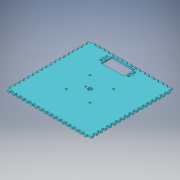
# Autodesk Inventor part: 000.206 - Крышка
Saved by Autodesk Inventor 2019 (Build 230136000, 136)
## iProperties
Created: 2020-02-27
Part Number: 000.206 - Крышка
Material: Типовые
Document SubType Name: Modeling
Designer: Петров Иван
Density: 1 g/cm^3
Appearance: Серо-синий
Author: Петров Иван
Autodesk Inventor part; units mm, degrees
ref_plane "YZ Plane" through (0, 0, 0) normal (1, 0, 0) x (0, 1, 0)
ref_plane "XZ Plane" through (0, 0, 0) normal (0, 1, 0) x (-1, 0, 0)
ref_plane "XY Plane" through (0, 0, 0) normal (0, 0, 1) x (1, 0, 0)
sketch "Эскиз1" plane through (0, 0, 0) normal (0, 1, 0) x (-1, 0, 0)
  line L0 (-72, 72) -> (72, 72)
  line L1 (72, 72) -> (72, -72)
  line L2 (72, -72) -> (-72, -72)
  line L3 (-72, -72) -> (-72, 72)
  line L4 (-72, 72) -> (72, -72) construction
  line L5 (72, 72) -> (-72, -72) construction
  point P0 (0, 0)
  dimension "d0" = 144
  dimension "d1" = 144
  constraints: 12 end point, 2 midpoint, 2 parallel, 1 horizontal, 1 perpendicular
  measures "d0" distance of L1.end L2.end
  measures "d1" distance of L0.end L1.end
extrude "Выдавливание1" add sketch "Эскиз1" along normal blind 3
sketch "Эскиз2" plane through (0, 3, 0) normal (0, 1, 0) x (1, 0, 0)
  line L0 (-72, 72) -> (-72, -72) projected
  line L1 (-72, -72) -> (-68, -72)
  line L2 (-68, -72) -> (-68, -75)
  line L3 (-68, -75) -> (-72, -75)
  line L4 (-72, -75) -> (-72, -72)
  point P0 (0, 0)
  dimension "d5" = 4
  dimension "d6" = 3
  constraints: 8 end point, 2 parallel, 1 horizontal, 1 perpendicular
  measures "d5" distance of L2.end L3.end
  measures "d6" distance of L1.end L2.end
extrude "Выдавливание2" add sketch "Эскиз2" against normal blind 3
pattern_linear "Прямоуг.массив1" count 18 spacing 8 along (1, 0, 0) of "Выдавливание2"
pattern_circular "Круговой массив1" count 4 over 360 about axis through (0, -10, 0) along (0, 1, 0) of "Выдавливание2", "Прямоуг.массив1"
sketch "Эскиз5" plane through (0, 3, 0) normal (0, 1, 0) x (1, 0, 0)
  line L0 (-37.7, 63.75) -> (-37.7, 60.5)
  line L1 (-37.7, 60.5) -> (-30.7, 60.5)
  line L2 (-30.7, 60.5) -> (-30.7, 70)
  line L3 (-30.7, 70) -> (-36.7, 70)
  arc A0 (-36.7, 70) -> (-37.7, 69) centre (-36.7, 69) ccw
  line L4 (-37.7, 69) -> (-37.7, 66.15)
  line L5 (-37.7, 66.15) -> (-36.634, 66.15)
  arc A1 (-36.634, 63.75) -> (-36.634, 66.15) centre (-34.85, 64.95) ccw
  line L6 (-36.634, 63.75) -> (-37.7, 63.75)
  line L7 (-37.7, 59.5) -> (-30.7, 59.5)
  line L8 (-37.7, 59.5) -> (-37.7, 56.25)
  line L9 (-37.7, 56.25) -> (-36.634, 56.25)
  arc A2 (-36.634, 53.85) -> (-36.634, 56.25) centre (-34.85, 55.05) ccw
  line L10 (-36.634, 53.85) -> (-37.7, 53.85)
  line L11 (-37.7, 53.85) -> (-37.7, 51)
  arc A3 (-37.7, 51) -> (-36.7, 50) centre (-36.7, 51) ccw
  line L12 (-36.7, 50) -> (-30.7, 50)
  line L13 (-30.7, 50) -> (-30.7, 59.5)
  line L14 (-37.7, 60.5) -> (-37.7, 59.5)
  line L15 (17, 60.5) -> (17, 59.5)
  line L16 (10, 59.5) -> (17, 59.5)
  line L17 (10, 50) -> (10, 59.5)
  line L18 (16, 50) -> (10, 50)
  arc A4 (16, 50) -> (17, 51) centre (16, 51) ccw
  line L19 (17, 53.85) -> (17, 51)
  line L20 (15.934, 53.85) -> (17, 53.85)
  arc A5 (15.934, 56.25) -> (15.934, 53.85) centre (14.15, 55.05) ccw
  line L21 (17, 56.25) -> (15.934, 56.25)
  line L22 (17, 59.5) -> (17, 56.25)
  line L23 (10, 60.5) -> (10, 70)
  line L24 (10, 60.5) -> (17, 60.5)
  line L25 (17, 63.75) -> (17, 60.5)
  line L26 (15.934, 63.75) -> (17, 63.75)
  arc A6 (15.934, 66.15) -> (15.934, 63.75) centre (14.15, 64.95) ccw
  line L27 (17, 66.15) -> (15.934, 66.15)
  line L28 (17, 69) -> (17, 66.15)
  arc A7 (17, 69) -> (16, 70) centre (16, 69) ccw
  line L29 (10, 70) -> (16, 70)
  line L30 (0, 70) -> (10, 70)
  line L31 (-30.7, 70) -> (0, 70)
  line L32 (-30.7, 50) -> (0, 50)
  line L33 (0, 50) -> (10, 50)
  circle A8 centre (0, 60) radius 5.4
  circle A9 centre (0, 60) radius 6.5
  circle A10 centre (0, 60) radius 1.25
  circle A11 centre (-34.85, 55.05) radius 2.15
  circle A12 centre (-34.85, 64.95) radius 2.15
  circle A13 centre (14.15, 64.95) radius 2.15
  circle A14 centre (14.15, 55.05) radius 2.15
  line L34 (15.934, 53.85) -> (17, 53.85)
  line L35 (17, 56.25) -> (15.934, 56.25)
  line L36 (17, 53.85) -> (17, 56.25)
  line L37 (17, 56.25) -> (17, 66.15)
  line L38 (17, 66.15) -> (15.934, 66.15)
  line L39 (17, 63.75) -> (17, 66.15)
  line L40 (-37.7, 63.75) -> (-37.7, 56.25)
  line L41 (-37.7, 66.15) -> (-37.7, 63.75)
  line L42 (-37.7, 56.25) -> (-36.634, 56.25)
  line L43 (-37.7, 56.25) -> (-37.7, 53.85)
  line L44 (0, 0) -> (0, 70)
  point P0 (-10.35, 50)
  dimension "d29" = 70
  constraints: 90 end point, 16 point on circle, 15 centre point, 4 coincident, 4 vertical, 3 concentric, 1 collinear, 1 perpendicular
  measures "d29" distance of L44.start L44.end
extrude "Выдавливание5" cut sketch "Эскиз5" against normal blind 10 contours L1 L2 L31 L44 A9 L32 L13 L7 L14 | A12 A1 | L30 L23 L24 L15 L16 L17 L33 L44 A9 | A2 A11 | L44 A8 A9 | A9 L44 A8 | L44 A10 A8 | A8 L44 A10 | L44 A10 | A10 L44 | A6 A13 | A14 A5
sketch "Эскиз6" plane through (0, 3, 0) normal (0, 1, 0) x (1, 0, 0)
  arc A0 (-18, 26.5) -> (-26.5, 18) centre (-18, 18) ccw
  line L0 (-26.5, -18) -> (-26.5, 18)
  arc A1 (-26.5, -18) -> (-18, -26.5) centre (-18, -18) ccw
  line L1 (18, -26.5) -> (-18, -26.5)
  arc A2 (18, -26.5) -> (26.5, -18) centre (18, -18) ccw
  line L2 (26.5, 18) -> (26.5, -18)
  arc A3 (26.5, 18) -> (18, 26.5) centre (18, 18) ccw
  line L3 (-18, 26.5) -> (18, 26.5)
  circle A4 centre (-21.2132, 21.2132) radius 1.5
  circle A5 centre (-21.2132, -21.2132) radius 1.5
  circle A6 centre (21.2132, -21.2132) radius 1.5
  circle A7 centre (21.2132, 21.2132) radius 1.5
  circle A8 centre (0, 0) radius 22
  constraints: 9 centre point, 8 end point, 8 point on circle
extrude "Выдавливание6" cut sketch "Эскиз6" against normal blind 10 contours A4 | A5 | A6 | A7
sketch "Эскиз7" plane through (0, 3, 0) normal (0, 1, 0) x (1, 0, 0)
  circle A0 centre (0, 0) radius 5.375
  circle A1 centre (0, 0) radius 3.375
  line L0 (-6.9327, -1) -> (-6.9327, 1)
  line L1 (-6.9327, 1) -> (-6.9327, 1.5)
  line L2 (-8.2327, 1.5) -> (-6.9327, 1.5)
  spline S0 degree 3 poles (-8.308, 1) (-8.3, 1.0653) (-8.2914, 1.1299) (-8.274, 1.2508) (-8.2654, 1.3061) (-8.2506, 1.3973) (-8.2444, 1.4332) (-8.2376, 1.4723) (-8.2358, 1.4829) (-8.2345, 1.49) (-8.2345, 1.4901) (-8.2345, 1.4902) (-8.2339, 1.4935) (-8.2333, 1.4967) (-8.2327, 1.5) knots 0 0 0 0 0.265855 0.265855 0.533308 0.533308 0.789424 0.789424 0.930547 0.930547 0.932946 0.932946 0.932946 1 1 1 1
  ellipse E0 centre (-0.8138, 2.2378) end of major axis (-6.2384, -4.8493) minor radius 6.6293 (-8.308, 1) -> (-8.3138, -1) ccw
  line L3 (-6.9327, -1.5) -> (-8.2327, -1.5)
  line L4 (-6.9327, -1.5) -> (-6.9327, -1)
  spline S1 degree 3 poles (-8.2327, -1.5) (-8.2334, -1.4968) (-8.234, -1.4935) (-8.2347, -1.4903) (-8.2347, -1.4901) (-8.2347, -1.49) (-8.2361, -1.4829) (-8.2382, -1.4724) (-8.2457, -1.4333) (-8.2525, -1.3974) (-8.2687, -1.3062) (-8.278, -1.2509) (-8.2965, -1.1299) (-8.3056, -1.0653) (-8.3138, -1) knots 0 0 0 0 0.066869 0.066869 0.066869 0.069411 0.069411 0.210348 0.210348 0.466356 0.466356 0.734146 0.734146 1 1 1 1
  line L5 (2.8341, 0.75) -> (-2.8341, 0.75)
  line L6 (2.8929, 0.7945) -> (2.8341, 0.75)
  arc A2 (2.8929, 0.7945) -> (2.8468, 0.9465) centre (0, 0) ccw
  line L7 (2.3559, 0.9758) -> (2.8468, 0.9465)
  line L8 (2.6823, 1.3437) -> (2.3559, 0.9758)
  arc A3 (2.6823, 1.3437) -> (2.6074, 1.4837) centre (0, 0) ccw
  line L9 (2.1202, 1.4167) -> (2.6074, 1.4837)
  line L10 (2.3686, 1.8411) -> (2.1202, 1.4167)
  arc A4 (2.3686, 1.8411) -> (2.2678, 1.9639) centre (0, 0) ccw
  line L11 (1.8031, 1.8031) -> (2.2678, 1.9639)
  line L12 (1.9639, 2.2678) -> (1.8031, 1.8031)
  arc A5 (1.9639, 2.2678) -> (1.8411, 2.3686) centre (0, 0) ccw
  line L13 (1.4167, 2.1202) -> (1.8411, 2.3686)
  line L14 (1.4837, 2.6074) -> (1.4167, 2.1202)
  arc A6 (1.4837, 2.6074) -> (1.3437, 2.6823) centre (0, 0) ccw
  line L15 (0.9758, 2.3559) -> (1.3437, 2.6823)
  line L16 (0.9465, 2.8468) -> (0.9758, 2.3559)
  arc A7 (0.9465, 2.8468) -> (0.7945, 2.8929) centre (0, 0) ccw
  line L17 (0.4975, 2.501) -> (0.7945, 2.8929)
  line L18 (0.373, 2.9767) -> (0.4975, 2.501)
  arc A8 (0.373, 2.9767) -> (0.2149, 2.9923) centre (0, 0) ccw
  line L19 (0, 2.55) -> (0.2149, 2.9923)
  line L20 (-0.2149, 2.9923) -> (0, 2.55)
  arc A9 (-0.2149, 2.9923) -> (-0.373, 2.9767) centre (0, 0) ccw
  line L21 (-0.4975, 2.501) -> (-0.373, 2.9767)
  line L22 (-0.7945, 2.8929) -> (-0.4975, 2.501)
  arc A10 (-0.7945, 2.8929) -> (-0.9465, 2.8468) centre (0, 0) ccw
  line L23 (-0.9758, 2.3559) -> (-0.9465, 2.8468)
  line L24 (-1.3437, 2.6823) -> (-0.9758, 2.3559)
  arc A11 (-1.3437, 2.6823) -> (-1.4837, 2.6074) centre (0, 0) ccw
  line L25 (-1.4167, 2.1202) -> (-1.4837, 2.6074)
  line L26 (-1.8411, 2.3686) -> (-1.4167, 2.1202)
  arc A12 (-1.8411, 2.3686) -> (-1.9639, 2.2678) centre (0, 0) ccw
  line L27 (-1.8031, 1.8031) -> (-1.9639, 2.2678)
  line L28 (-2.2678, 1.9639) -> (-1.8031, 1.8031)
  arc A13 (-2.2678, 1.9639) -> (-2.3686, 1.8411) centre (0, 0) ccw
  line L29 (-2.1202, 1.4167) -> (-2.3686, 1.8411)
  line L30 (-2.6074, 1.4837) -> (-2.1202, 1.4167)
  arc A14 (-2.6074, 1.4837) -> (-2.6823, 1.3437) centre (0, 0) ccw
  line L31 (-2.3559, 0.9758) -> (-2.6823, 1.3437)
  line L32 (-2.8468, 0.9465) -> (-2.3559, 0.9758)
  arc A15 (-2.8468, 0.9465) -> (-2.8929, 0.7945) centre (0, 0) ccw
  line L33 (-2.8341, 0.75) -> (-2.8929, 0.7945)
  arc A16 (-2.8929, 0.7945) -> (-2.8929, -0.7945) centre (0, 0) ccw
  line L34 (2.8929, 0.7945) -> (2.8341, 0.75)
  line L35 (2.8341, 0.75) -> (-2.8341, 0.75)
  line L36 (-2.8341, 0.75) -> (-2.8929, 0.7945)
  arc A17 (-2.8929, 0.7945) -> (-2.8929, -0.7945) centre (0, 0) ccw
  line L37 (-2.8929, -0.7945) -> (-2.8341, -0.75)
  line L38 (-2.8341, -0.75) -> (2.8341, -0.75)
  line L39 (2.8341, -0.75) -> (2.8929, -0.7945)
  arc A18 (2.8929, -0.7945) -> (2.8929, 0.7945) centre (0, 0) ccw
  line L40 (-2.8341, -0.75) -> (2.8341, -0.75)
  line L41 (-2.8929, -0.7945) -> (-2.8341, -0.75)
  arc A19 (-2.8929, -0.7945) -> (-2.8468, -0.9465) centre (0, 0) ccw
  line L42 (-2.3559, -0.9758) -> (-2.8468, -0.9465)
  line L43 (-2.6823, -1.3437) -> (-2.3559, -0.9758)
  arc A20 (-2.6823, -1.3437) -> (-2.6074, -1.4837) centre (0, 0) ccw
  line L44 (-2.1202, -1.4167) -> (-2.6074, -1.4837)
  line L45 (-2.3686, -1.8411) -> (-2.1202, -1.4167)
  arc A21 (-2.3686, -1.8411) -> (-2.2678, -1.9639) centre (0, 0) ccw
  line L46 (-1.8031, -1.8031) -> (-2.2678, -1.9639)
  line L47 (-1.9639, -2.2678) -> (-1.8031, -1.8031)
  arc A22 (-1.9639, -2.2678) -> (-1.8411, -2.3686) centre (0, 0) ccw
  line L48 (-1.4167, -2.1202) -> (-1.8411, -2.3686)
  line L49 (-1.4837, -2.6074) -> (-1.4167, -2.1202)
  arc A23 (-1.4837, -2.6074) -> (-1.3437, -2.6823) centre (0, 0) ccw
  line L50 (-0.9758, -2.3559) -> (-1.3437, -2.6823)
  line L51 (-0.9465, -2.8468) -> (-0.9758, -2.3559)
  arc A24 (-0.9465, -2.8468) -> (-0.7945, -2.8929) centre (0, 0) ccw
  line L52 (-0.4975, -2.501) -> (-0.7945, -2.8929)
  line L53 (-0.373, -2.9767) -> (-0.4975, -2.501)
  arc A25 (-0.373, -2.9767) -> (-0.2149, -2.9923) centre (0, 0) ccw
  line L54 (0, -2.55) -> (-0.2149, -2.9923)
  line L55 (0.2149, -2.9923) -> (0, -2.55)
  arc A26 (0.2149, -2.9923) -> (0.373, -2.9767) centre (0, 0) ccw
  line L56 (0.4975, -2.501) -> (0.373, -2.9767)
  line L57 (0.7945, -2.8929) -> (0.4975, -2.501)
  arc A27 (0.7945, -2.8929) -> (0.9465, -2.8468) centre (0, 0) ccw
  line L58 (0.9758, -2.3559) -> (0.9465, -2.8468)
  line L59 (1.3437, -2.6823) -> (0.9758, -2.3559)
  arc A28 (1.3437, -2.6823) -> (1.4837, -2.6074) centre (0, 0) ccw
  line L60 (1.4167, -2.1202) -> (1.4837, -2.6074)
  line L61 (1.8411, -2.3686) -> (1.4167, -2.1202)
  arc A29 (1.8411, -2.3686) -> (1.9639, -2.2678) centre (0, 0) ccw
  line L62 (1.8031, -1.8031) -> (1.9639, -2.2678)
  line L63 (2.2678, -1.9639) -> (1.8031, -1.8031)
  arc A30 (2.2678, -1.9639) -> (2.3686, -1.8411) centre (0, 0) ccw
  line L64 (2.1202, -1.4167) -> (2.3686, -1.8411)
  line L65 (2.6074, -1.4837) -> (2.1202, -1.4167)
  arc A31 (2.6074, -1.4837) -> (2.6823, -1.3437) centre (0, 0) ccw
  line L66 (2.3559, -0.9758) -> (2.6823, -1.3437)
  line L67 (2.8468, -0.9465) -> (2.3559, -0.9758)
  arc A32 (2.8468, -0.9465) -> (2.8929, -0.7945) centre (0, 0) ccw
  line L68 (2.8341, -0.75) -> (2.8929, -0.7945)
  constraints: 138 end point, 62 point on circle, 33 centre point, 8 other
extrude "Выдавливание7" cut sketch "Эскиз7" against normal blind 10 contours A1 | L4 L3 S1 E0 S0 L2 L1 L0 | L6 A18 L39 L38 L37 A16 L33 L5 | L5 L33 A15 L32 L31 A14 L30 L29 A13 L28 L27 A12 L26 L25 A11 L24 L23 A10 L22 L21 A9 L20 L19 A8 L18 L17 A7 L16 L15 A6 L14 L13 A5 L12 L11 A4 L10 L9 A3 L8 L7 A2 L6 | A32 L67 L66 A31 L65 L64 A30 L63 L62 A29 L61 L60 A28 L59 L58 A27 L57 L56 A26 L55 L54 A25 L53 L52 A24 L51 L50 A23 L49 L48 A22 L47 L46 A21 L45 L44 A20 L43 L42 A19 L37 L38 L39
sketch "Эскиз8" plane through (0, 3, 0) normal (0, 1, 0) x (1, 0, 0)
  circle A0 centre (-67.69, 17.6749) radius 3 projected
  line L0 (-65.15, 32.4749) -> (-65.15, 45.8749) projected
  line L1 (-68.6559, 43.7249) -> (-68.6559, 34.6249) projected
  line L2 (-70.0861, 59.3712) -> (-70.0861, 61.7787) projected
  line L3 (-69.0955, 58.7249) -> (-69.0955, 62.4249) projected
  line L4 (-75, 4) -> (-75, 8) projected
  line L5 (-55, 68) -> (-75, 68)
  line L6 (-75, 68) -> (-75, 8)
  line L7 (-75, 8) -> (-55, 8)
  line L8 (-55, 8) -> (-55, 68)
  line L9 (-75, 64) -> (-72, 64) projected
  line L10 (-72, 68) -> (-75, 68) projected
  point P0 (0, 0)
  dimension "d33" = 20
  dimension "d36" = 0
  constraints: 8 end point, 2 parallel, 1 horizontal, 1 perpendicular
  measures "d33" distance between parallel lines of L8 L6
  measures "d36" distance between parallel lines of L10 L5
extrude "Выдавливание8" [suppressed]
